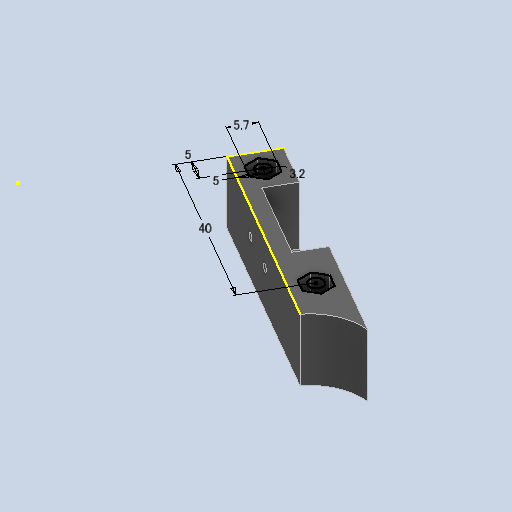
# Autodesk Inventor part: limit_setter_under
Saved by Autodesk Inventor 2024.1 (Build 281209000, 209)
## iProperties
Created: 2025-01-18
Part Number: limit_setter_under
Material: 一般
Document SubType Name: Modeling
Designer: hibik
Density: 1 g/cm^3
Appearance: 既定
Author: hibik
Autodesk Inventor part; units mm, degrees
ref_plane "YZ Plane" through (0, 0, 0) normal (1, 0, 0) x (0, 1, 0)
ref_plane "XZ Plane" through (0, 0, 0) normal (0, 1, 0) x (-1, 0, 0)
ref_plane "XY Plane" through (0, 0, 0) normal (0, 0, 1) x (1, 0, 0)
sketch "スケッチ1" plane through (0, 0, 0) normal (0, 1, 0) x (-1, 0, 0)
  line L0 (0, 0) -> (0, -40)
  line L1 (0, -40) -> (-23.7735, -40)
  line L2 (-23.7735, -40) -> (-54.0844, -22.5)
  line L3 (0, -30) -> (-18, -30)
  line L4 (-18, -30) -> (-38, -18.453)
  line L5 (-28, -24.2265) -> (-28, 11.9512)
  line L6 (-18, -30) -> (-23.7735, -40)
  line L7 (-18.7735, -31.3397) -> (-20.74, -30.2044)
  line L8 (-20.74, -30.2044) -> (-58.951, -8.1433)
  line L9 (-33.7735, -34.2265) -> (-30.4735, -28.5107)
  line L10 (-30.4735, -28.5107) -> (-47.5342, -18.6607)
  line L11 (-47.5342, -18.6607) -> (-50.8342, -24.3765)
  line L12 (-50.8342, -24.3765) -> (-33.7735, -34.2265)
  line L13 (-30.4735, -28.5107) -> (-28, -24.2265)
  line L14 (-24.6395, -39.5) -> (-19.5508, -30.686)
  line L15 (-54.0844, -22.5) -> (-49.0844, -13.8397)
  point P0 (-19.6395, -30.8397)
  dimension "d0" = 40
  dimension "d1" = 30
  dimension "d2" = 18
  dimension "d3" = 30
  dimension "d4" = 38
  dimension "d5" = 10
  dimension "d6" = 10
  dimension "d7" = 19.7
  dimension "d8" = 6.6
  dimension "d9" = 1
  dimension "d10" = 35
  constraints: 32 end point, 6 perpendicular, 5 parallel, 4 point on line, 2 horizontal, 2 midpoint, 2 vertical, 1 collinear
  measures "d0" distance of L0.start L0.end
  measures "d1" angle of L1 L2
  measures "d2" distance of L3.start L3.end
  measures "d3" distance of L0.start L3.start
  measures "d4" distance from line of L0 L4.end
  measures "d5" distance from line of L3.end L5
  measures "d6" distance between parallel lines of L2 L8
  measures "d7" distance between parallel lines of L11 L9
  measures "d8" distance between parallel lines of L12 L10
  measures "d9" distance between parallel lines of L6 L14
  measures "d10" distance between parallel lines of L15 L6
extrude "押し出し1" add sketch "スケッチ1" along normal blind 15 contours L2 L9 L13 L8 L7 L14 | L13 L10 L11 L2 L15 L8
sketch "スケッチ2" plane through (0, 0, 0) normal (0, -1, 0) x (1, 0, 0)
  line L0 (30.4735, -28.5107) -> (33.7735, -34.2265) projected
  line L1 (47.5342, -18.6607) -> (30.4735, -28.5107) projected
  line L2 (50.8342, -24.3765) -> (47.5342, -18.6607) projected
  line L3 (54.0844, -22.5) -> (50.8342, -24.3765) projected
  line L4 (49.0844, -13.8397) -> (54.0844, -22.5) projected
  line L5 (19.6395, -30.8397) -> (49.0844, -13.8397) projected
  line L6 (24.6395, -39.5) -> (19.6395, -30.8397) projected
  line L7 (33.7735, -34.2265) -> (24.6395, -39.5) projected
  line L8 (50.8342, -24.3765) -> (33.7735, -34.2265)
  point P0 (0, 0)
  constraints: 2 end point
extrude "押し出し2" add sketch "スケッチ2" against normal blind 1
sketch "スケッチ3" plane through (30.4735, 1, -28.5107) normal (0.5, 0, -0.8660254) x (-0.8660254, 0, -0.5)
  line L0 (-19.7, 0) -> (0, 0) projected
  line L1 (-19.7, 14) -> (0, 14) projected
  line L2 (-9.85, 14) -> (-9.85, 0)
  line L3 (-19.7, 0) -> (0, 0) projected
  circle A0 centre (-14.6, 7.9) radius 0.85
  circle A1 centre (-5.1, 7.9) radius 0.85
  point P0 (12.1355, -1)
  dimension "d16" = 1.7
  dimension "d17" = 9.5
  dimension "d18" = 7.9
  constraints: 2 centre point, 2 end point, 2 midpoint, 1 equal radius, 1 symmetric about line
  measures "d16" diameter of A1
  measures "d17" distance of A0.centre A1.centre
  measures "d18" distance from line of L0 A1.centre
extrude "押し出し3" cut sketch "スケッチ3" against normal through all
sketch "スケッチ4" plane through (0, 0, 0) normal (0, -1, 0) x (1, 0, 0)
  circle A0 centre (50.5, 0) radius 1.5 projected
  circle A1 centre (50.5, 0) radius 12.5
  line L0 (49.0844, -13.8397) -> (54.0844, -22.5) projected
  line L1 (49.0844, -13.8397) -> (54.0844, -22.5)
  line L2 (54.0844, -22.5) -> (74.7158, -10.5885)
  line L3 (74.7158, -10.5885) -> (69.7158, -1.9282)
  line L4 (69.7158, -1.9282) -> (49.0844, -13.8397)
  line L5 (74.7158, -10.5885) -> (86.6025, 10) projected
  circle A2 centre (71.4838, 0.8246) radius 1.5 projected
  circle A3 centre (71.4838, 0.8246) radius 12.5
  point P0 (0, 0)
  point P1 (60.8076, -7.0714)
  point P2 (51.4702, -12.4623)
  point P3 (72.3273, -6.4515)
  point P4 (61.4867, -6.6793)
  point P5 (72.9912, -11.5842)
  dimension "d21" = 25
  dimension "d24" = 25
  constraints: 8 end point, 3 equal length, 2 centre point, 2 coincident, 1 perpendicular, 1 point on line
  measures "d21" diameter of A1
  measures "d24" diameter of A3
extrude "押し出し4" add sketch "スケッチ4" against normal up to surface (15 mm away) contours L4 A1 | A1 L4 A3 L2 L0
sketch "スケッチ5" plane through (0, 15, 0) normal (0, 1, 0) x (1, 0, 0)
  line L0 (56.7805, 18.4608) -> (59.6305, 16.8153)
  line L1 (59.6305, 16.8153) -> (59.6305, 13.5244)
  line L2 (59.6305, 13.5244) -> (56.7805, 11.879)
  line L3 (56.7805, 11.879) -> (53.9305, 13.5244)
  line L4 (53.9305, 13.5244) -> (53.9305, 16.8153)
  line L5 (53.9305, 16.8153) -> (56.7805, 18.4608)
  line L6 (26.4697, 35.9608) -> (29.3197, 34.3153)
  line L7 (29.3197, 34.3153) -> (29.3197, 31.0244)
  line L8 (29.3197, 31.0244) -> (26.4697, 29.379)
  line L9 (26.4697, 29.379) -> (23.6197, 31.0244)
  line L10 (23.6197, 31.0244) -> (23.6197, 34.3153)
  line L11 (23.6197, 34.3153) -> (26.4697, 35.9608)
  line L12 (19.6395, 30.8397) -> (61.4867, 6.6793) projected
  line L13 (24.6395, 39.5) -> (19.6395, 30.8397) projected
  circle A0 centre (56.7805, 15.1699) radius 1.6
  circle A1 centre (26.4697, 32.6699) radius 1.6
  point P0 (0, 0)
  dimension "d25" = 5.7
  dimension "d26" = 5
  dimension "d27" = 5
  dimension "d28" = 40
  dimension "d29" = 3.2
  constraints: 24 end point, 2 centre point, 2 coincident, 2 collinear, 2 parallel, 1 equal radius, 26 other
  measures "d25" distance between parallel lines of L6 L9
  measures "d26" distance from line of L12 point (26.47, 32.67)
  measures "d27" distance from line of point (26.47, 32.67) L13
  measures "d28" distance from line of point (56.781, 15.17) L13
  measures "d29" diameter of A1
extrude "押し出し5" cut sketch "スケッチ5" against normal blind 10 contours L0 L1 L2 L3 L4 L5 | L6 L7 L8 L9 L10 L11 | A0 | A1
extrude "押し出し6" cut sketch "スケッチ5" against normal through all contours A0 | A1
